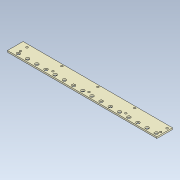
# Autodesk Inventor part: top_cover_02
Saved by Autodesk Inventor 2022.4 (Build 264492010, 492A)
## iProperties
Created: 2023-04-17
Part Number: top_cover_02
Material: Generic
Document SubType Name: Modeling
Designer: SB13FLLT004
Density: 1 g/cm^3
Appearance: Yellow(1)
Author: SB13FLLT004
Autodesk Inventor part; units mm, degrees
ref_plane "YZ Plane" through (0, 0, 0) normal (1, 0, 0) x (0, 1, 0)
ref_plane "XZ Plane" through (0, 0, 0) normal (0, 1, 0) x (-1, 0, 0)
ref_plane "XY Plane" through (0, 0, 0) normal (0, 0, 1) x (1, 0, 0)
derived "main_manifold_8v_v02.ipt"
sketch "Sketch:MM: prop valve cutout" plane through (0, 0, 0) normal (1, 0, 0) x (0, 1, 0)
  line L0 (20.32, -27.94) -> (20.32, 0)
  line L1 (0, -27.94) -> (20.32, -27.94)
  line L2 (20.32, -25.781) -> (16.256, -25.781)
  line L3 (16.256, -25.781) -> (16.256, -27.94)
  point P0 (0, 0)
  point P1 (12.5222, -27.94)
sketch "Sketch:MM: MMC screws" plane through (0, 20.32, 0) normal (0, 1, 0) x (1, 0, 0)
  line L0 (0, 0) -> (0, 27.94)
  line L1 (43.815, 4.699) -> (59.055, 4.699) construction
  line L2 (0, 0) -> (247.65, 0)
  line L3 (13.335, 4.699) -> (28.575, 4.699) construction
  line L4 (74.295, 4.699) -> (89.535, 4.699) construction
  line L5 (104.775, 4.699) -> (120.015, 4.699) construction
  line L6 (135.255, 4.699) -> (150.495, 4.699) construction
  line L7 (165.735, 4.699) -> (180.975, 4.699) construction
  line L8 (196.215, 4.699) -> (211.455, 4.699) construction
  line L9 (226.695, 4.699) -> (241.935, 4.699) construction
  point P0 (20.955, 4.699)
  point P1 (112.395, 4.699)
  point P2 (51.435, 4.699)
  point P3 (81.915, 4.699)
  point P4 (0, 25.781)
  point P5 (0, 25.781)
  point P6 (0, 25.781)
  point P7 (142.875, 4.699)
  point P8 (173.355, 4.699)
  point P9 (203.835, 4.699)
  point P10 (234.315, 4.699)
  point P11 (20.955, 4.699)
  point P12 (51.435, 4.699)
  point P13 (81.915, 4.699)
  point P14 (112.395, 4.699)
  point P15 (142.875, 4.699)
  point P16 (173.355, 4.699)
  point P17 (203.835, 4.699)
  point P18 (234.315, 4.699)
sketch "Sketch:MM: bath & TC screws" plane through (0, 20.32, 0) normal (0, 1, 0) x (1, 0, 0)
  arc A0 (17.78, 17.1704) -> (17.78, 13.3096) centre (17.78, 15.24) ccw
  arc A1 (237.49, 13.3096) -> (237.49, 17.1704) centre (237.49, 15.24) ccw
  line L0 (17.78, 13.3096) -> (237.49, 13.3096)
  line L1 (17.78, 17.1704) -> (237.49, 17.1704)
  arc A2 (17.78, 17.8054) -> (17.78, 12.6746) centre (17.78, 15.24) ccw
  arc A3 (237.49, 12.6746) -> (237.49, 17.8054) centre (237.49, 15.24) ccw
  line L2 (17.78, 12.6746) -> (237.49, 12.6746)
  line L3 (17.78, 17.8054) -> (237.49, 17.8054)
  arc A4 (17.78, 19.939) -> (17.78, 10.541) centre (17.78, 15.24) ccw
  arc A5 (237.49, 10.541) -> (237.49, 19.939) centre (237.49, 15.24) ccw
  line L4 (237.49, 19.939) -> (17.78, 19.939)
  line L5 (237.49, 10.541) -> (17.78, 10.541)
  line L6 (0, 27.94) -> (247.65, 27.94)
  line L7 (11.557, 20.701) -> (11.557, 9.779) construction
  line L8 (67.437, 22.606) -> (67.437, 7.874) construction
  circle A6 centre (11.557, 20.701) radius 1.6383 construction
  circle A7 centre (11.557, 9.779) radius 1.6383 construction
  circle A8 centre (243.967, 20.701) radius 1.6383 construction
  circle A9 centre (243.967, 9.779) radius 1.6383 construction
  point P0 (0, 0)
  point P1 (20.955, 27.94)
  point P2 (234.315, 27.94)
  point P3 (127.127, 22.606)
  point P4 (127.127, 7.874)
  point P5 (188.087, 22.606)
  point P6 (188.087, 7.874)
  point P7 (11.557, 15.24)
  point P8 (11.557, 15.24)
  point P9 (67.437, 15.24)
  point P10 (67.437, 15.24)
  point P11 (0, 15.24)
sketch "TC: base" plane through (0, 0, 0) normal (0, 1, 0) x (-1, 0, 0)
  line L0 (0, -25.781) -> (-247.65, -25.781)
  line L1 (-247.65, -25.781) -> (-247.65, 0)
  line L2 (-247.65, 0) -> (0, 0)
  line L3 (0, 0) -> (0, -25.781)
  line L4 (0, -25.781) -> (0, -27.94) construction
  line L5 (0, -27.94) -> (0, 0) construction
  constraints: 8 end point, 3 perpendicular, 1 horizontal, 1 horizontal alignment
extrude "Ex: base" add sketch "TC: base" along normal blind 2.54
hole "Hole: TC screws: 4-40 through hole" at (67.437, 20.32, -7.874) at (127.127, 20.32, -7.874) at (127.127, 20.32, -22.606) at (67.437, 20.32, -22.606) at (188.087, 20.32, -7.874) at (188.087, 20.32, -22.606) at (11.557, 20.32, -9.779) at (11.557, 20.32, -20.701) at (243.967, 20.32, -9.779) at (243.967, 20.32, -20.701) direction (0, -1, 0) diameter 3.2766 end through all clearance for "Socket Head Cap Screw" size "#4" standard "Ansi Unified Screw Threads"
hole "Hole: MMC screws: 4-40 head through hole" at (13.335, 20.32, -4.699) at (28.575, 20.32, -4.699) at (43.815, 20.32, -4.699) at (59.055, 20.32, -4.699) at (74.295, 20.32, -4.699) at (89.535, 20.32, -4.699) at (104.775, 20.32, -4.699) at (120.015, 20.32, -4.699) at (135.255, 20.32, -4.699) at (150.495, 20.32, -4.699) at (165.735, 20.32, -4.699) at (180.975, 20.32, -4.699) at (196.215, 20.32, -4.699) at (211.455, 20.32, -4.699) at (226.695, 20.32, -4.699) at (241.935, 20.32, -4.699) direction (0, -1, 0) diameter 5.5626 end through all
body "Solid1"
